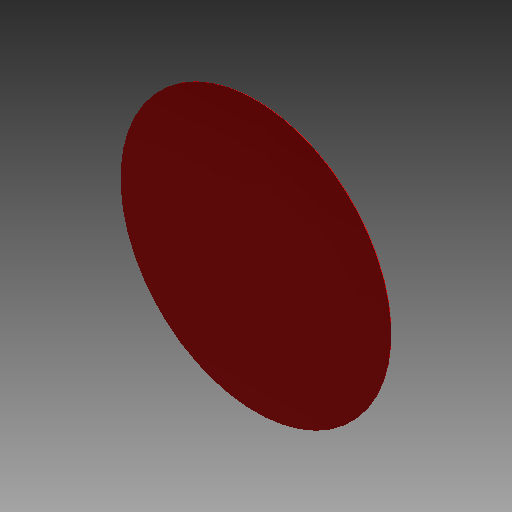
# Autodesk Inventor part: Hole
Saved by Autodesk Inventor 2018.2 (Build 222227000, 227)
## iProperties
Part Number: Hole
Material: Generic
Document SubType Name: Modeling
Designer: autocad
Appearance: Wave_hole_3x7-singleSided, Hole
Author: autocad
Autodesk Inventor part; units mm, degrees
ref_plane "YZ Plane" through (0, 0, 0) normal (1, 0, 0) x (0, 1, 0)
ref_plane "XZ Plane" through (0, 0, 0) normal (0, 1, 0) x (-1, 0, 0)
ref_plane "XY Plane" through (0, 0, 0) normal (0, 0, 1) x (1, 0, 0)
sketch "Wave_hole_3x7-singleSided, Hole_352" plane through (0, 0, 0) normal (0, 0, 1) x (1, 0, 0)
  line L0 (0.5213, 2.6209) -> (0.859, 2.5304)
  line L1 (0.859, 2.5304) -> (1.1819, 2.3966)
  line L2 (1.1819, 2.3966) -> (1.4846, 2.2219)
  line L3 (1.4846, 2.2219) -> (1.7619, 2.0091)
  line L4 (1.7619, 2.0091) -> (2.0091, 1.7619)
  line L5 (2.0091, 1.7619) -> (2.2219, 1.4846)
  line L6 (2.2219, 1.4846) -> (2.3966, 1.1819)
  line L7 (2.3966, 1.1819) -> (2.5304, 0.859)
  line L8 (2.5304, 0.859) -> (2.6209, 0.5213)
  line L9 (2.6209, 0.5213) -> (2.6665, 0.1748)
  line L10 (2.6665, 0.1748) -> (2.6665, 0)
  line L11 (2.6665, 0) -> (2.6665, -0.1748)
  line L12 (2.6665, -0.1748) -> (2.6209, -0.5213)
  line L13 (2.6209, -0.5213) -> (2.5304, -0.859)
  line L14 (2.5304, -0.859) -> (2.3966, -1.1819)
  line L15 (2.3966, -1.1819) -> (2.2219, -1.4846)
  line L16 (2.2219, -1.4846) -> (2.0091, -1.7619)
  line L17 (2.0091, -1.7619) -> (1.7619, -2.0091)
  line L18 (1.7619, -2.0091) -> (1.4846, -2.2219)
  line L19 (1.4846, -2.2219) -> (1.1819, -2.3966)
  line L20 (1.1819, -2.3966) -> (0.859, -2.5304)
  line L21 (0.859, -2.5304) -> (0.5213, -2.6209)
  line L22 (0.5213, -2.6209) -> (0.1748, -2.6665)
  line L23 (0.1748, -2.6665) -> (-0.1748, -2.6665)
  line L24 (-0.1748, -2.6665) -> (-0.5213, -2.6209)
  line L25 (-0.5213, -2.6209) -> (-0.859, -2.5304)
  line L26 (-0.859, -2.5304) -> (-1.1819, -2.3966)
  line L27 (-1.1819, -2.3966) -> (-1.4846, -2.2219)
  line L28 (-1.4846, -2.2219) -> (-1.7619, -2.0091)
  line L29 (-1.7619, -2.0091) -> (-2.0091, -1.7619)
  line L30 (-2.0091, -1.7619) -> (-2.2219, -1.4846)
  line L31 (-2.2219, -1.4846) -> (-2.3966, -1.1819)
  line L32 (-2.3966, -1.1819) -> (-2.5304, -0.859)
  line L33 (-2.5304, -0.859) -> (-2.6209, -0.5213)
  line L34 (-2.6209, -0.5213) -> (-2.6665, -0.1748)
  line L35 (-2.6665, -0.1748) -> (-2.6665, 0)
  line L36 (-2.6665, 0) -> (-2.6665, 0.1748)
  line L37 (-2.6665, 0.1748) -> (-2.6209, 0.5213)
  line L38 (-2.6209, 0.5213) -> (-2.5304, 0.859)
  line L39 (-2.5304, 0.859) -> (-2.3966, 1.1819)
  line L40 (-2.3966, 1.1819) -> (-2.2219, 1.4846)
  line L41 (-2.2219, 1.4846) -> (-2.0091, 1.7619)
  line L42 (-2.0091, 1.7619) -> (-1.7619, 2.0091)
  line L43 (-1.7619, 2.0091) -> (-1.4846, 2.2219)
  line L44 (-1.4846, 2.2219) -> (-1.1819, 2.3966)
  line L45 (-1.1819, 2.3966) -> (-0.859, 2.5304)
  line L46 (-0.859, 2.5304) -> (-0.5213, 2.6209)
  line L47 (-0.5213, 2.6209) -> (-0.1748, 2.6665)
  line L48 (-0.1748, 2.6665) -> (0.1748, 2.6665)
  line L49 (0.1748, 2.6665) -> (0.5213, 2.6209)
  constraints: 100 end point
extrude "Extrusion1" add sketch "Wave_hole_3x7-singleSided, Hole_352" along normal blind 0.01
body "Solid1"
